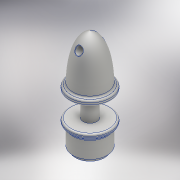
# Autodesk Inventor part: Prop Holder
Saved by Autodesk Inventor 2018 (Build 220112000, 112)
## iProperties
Created: 2018-01-07
Part Number: Prop Holder
Material: Aluminum 6061
Document SubType Name: Modeling
Designer: fbl92568
Density: 2.7 g/cm^3
Appearance: Aluminum - Flat
Author: fbl92568
Autodesk Inventor part; units mm, degrees
ref_plane "YZ Plane" through (0, 0, 0) normal (1, 0, 0) x (0, 1, 0)
ref_plane "XZ Plane" through (0, 0, 0) normal (0, 1, 0) x (-1, 0, 0)
ref_plane "XY Plane" through (0, 0, 0) normal (0, 0, 1) x (1, 0, 0)
sketch "Sketch1" plane through (0, 0, 0) normal (0, 0, 1) x (1, 0, 0)
  circle A0 centre (0, 0) radius 4.25
  dimension "d0" = 8.5
  constraints: 1 centre point, 1 coincident
  measures "d0" diameter of A0
extrude "Extrusion1" add sketch "Sketch1" along normal blind 1
sketch "Sketch2" plane through (0, 0, 1) normal (0, 0, 1) x (1, 0, 0)
  circle A0 centre (0, 0) radius 5
  dimension "d3" = 10
  constraints: 1 centre point, 1 coincident
  measures "d3" diameter of A0
extrude "Extrusion2" add sketch "Sketch2" along normal blind 5
sketch "Sketch3" plane through (0, 0, 6) normal (0, 0, 1) x (1, 0, 0)
  circle A0 centre (0, 0) radius 6
  dimension "d6" = 12
  constraints: 1 centre point, 1 coincident
  measures "d6" diameter of A0
extrude "Extrusion3" add sketch "Sketch3" along normal blind 2
chamfer "Chamfer1" distance 1 angle 45 1 edges at (-6, 0, 6)
sketch "Sketch4" plane through (0, 0, 8) normal (0, 0, 1) x (1, 0, 0)
  circle A0 centre (0, 0) radius 2
  dimension "d12" = 4
  constraints: 1 centre point, 1 coincident
  measures "d12" diameter of A0
extrude "Extrusion4" add sketch "Sketch4" along normal blind 7
sketch "Sketch5" plane through (0, 0, 15) normal (0, 0, 1) x (1, 0, 0)
  circle A0 centre (0, 0) radius 6
  dimension "d15" = 12
  constraints: 1 centre point, 1 coincident
  measures "d15" diameter of A0
extrude "Extrusion5" add sketch "Sketch5" along normal blind 1.5
sketch "Sketch6" plane through (0, 0, 0) normal (1, 0, 0) x (0, 1, 0)
  line L0 (-6, 15) -> (6, 15) projected
  line L1 (6, 16.5) -> (-6, 16.5) projected
  line L2 (5, 16.5) -> (0, 16.5)
  line L3 (0, 16.5) -> (0, 30)
  line L4 (5, 16.5) -> (5, 22.6463) construction
  line L5 (5, 22.6463) -> (3.7203, 28.7891) construction
  line L6 (3.7203, 28.7891) -> (0, 30) construction
  spline S0 degree 3 poles (5, 16.5) (5, 22.6463) (3.7203, 28.7891) (0, 30) knots 1 1 1 1 2 2 2 2
  point P0 (0, 0)
  dimension "d18" = 15
  dimension "d19" = 5
  constraints: 4 end point, 1 midpoint, 1 perpendicular, 1 point on line, 1 vertical, 3 other
  measures "d18" distance from line of L3.end L0
  measures "d19" distance from line of L3 L2.start
revolve "Revolution1" add sketch "Sketch6" angle 360 about axis through (0, 0, 16.5) along (0, 0, 1)
sketch "Sketch7" plane through (0, 0, 0) normal (0, 1, 0) x (-1, 0, 0)
  circle A0 centre (0, 26.5) radius 1
  line L0 (0, 16.5) -> (0, 30) projected
  line L1 (-5, 16.5) -> (5, 16.5) projected
  line L2 (6, 16.5) -> (-6, 16.5) projected
  point P0 (0, 0)
  dimension "d21" = 2
  dimension "d22" = 10
  constraints: 1 centre point
  measures "d21" diameter of A0
  measures "d22" distance from line of L2 A0.centre
extrude "Extrusion6" cut sketch "Sketch7" along normal through all both and the other way through all
fillet "Fillet1" radius 0.1 5 edges at (0.9868, -3.1395, 26.6619) (-0.9798, -3.3103, 26.2999) (-0.7241, 3.5759, 25.8103) (-0.7171, 2.9356, 27.1969) (0.9998, 3.223, 26.4786)
fillet "Fillet1" radius 0.5 7 edges at (0, -5, 16.5) (-6, 0, 16.5) (-6, 0, 15) (-6, 0, 8) (-6, 0, 6.9999) (-5.0001, 0, 6) (-5, 0, 6)
sketch "Sketch8" plane through (0, 0, 0) normal (0, 1, 0) x (-1, 0, 0)
  line L0 (-4.25, 0) -> (4.25, 0) projected
  line L1 (-4.25, 0) -> (-4.0245, 0.9885)
  line L2 (-4.0245, 0.9885) -> (-4.25, 1)
  line L3 (-5, 1) -> (5, 1) projected
  line L4 (-4.25, 0) -> (-4.25, 1)
  line L5 (-4.25, 0) -> (-4.25, 1) projected
  line L6 (0, -6) -> (0, 36) projected
  point P0 (0, 0)
  constraints: 6 end point, 1 collinear, 1 point on line
revolve "Revolution2" cut sketch "Sketch8" angle 360 about axis through (0, 0, -10) along (0, 0, 1) contours L4 L2 L1
sketch "Sketch9" plane through (0, 0, 0) normal (0, 0, -1) x (-1, 0, 0)
  circle A0 centre (0, 0) radius 1.5
  dimension "d28" = 3
  constraints: 1 centre point, 1 coincident
  measures "d28" diameter of A0
extrude "Extrusion7" cut sketch "Sketch9" against normal blind 10
body "Solid1"
